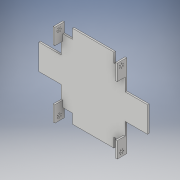
# Autodesk Inventor part: Gen2PlatePart
Saved by Autodesk Inventor 2017 (Build 210142000, 142)
## iProperties
Created: 2017-12-06
Part Number: Gen2PlatePart
Material: Generic
Document SubType Name: Modeling
Designer: User
Density: 1 g/cm^3
Appearance: Default
Author: User
Autodesk Inventor part; units mm, degrees
ref_plane "YZ Plane" through (0, 0, 0) normal (1, 0, 0) x (0, 1, 0)
ref_plane "XZ Plane" through (0, 0, 0) normal (0, 1, 0) x (-1, 0, 0)
ref_plane "XY Plane" through (0, 0, 0) normal (0, 0, 1) x (1, 0, 0)
sketch "Sketch1" plane through (0, 0, 0) normal (0, 0, 1) x (1, 0, 0)
  line L0 (0, 0) -> (254, 0)
  line L1 (254, 0) -> (254, 330.2)
  line L2 (254, 330.2) -> (0, 330.2)
  line L3 (0, 330.2) -> (0, 0)
  dimension "d0" = 254
  dimension "d1" = 330.2
  constraints: 8 end point, 2 parallel, 1 horizontal, 1 perpendicular
  measures "d0" distance of L2.end L1.end
  measures "d1" distance of L1.end L0.end
extrude "Extrusion1" add sketch "Sketch1" along normal blind 6.35
sketch "Sketch2" plane through (0, 0, 6.35) normal (0, 0, 1) x (1, 0, 0)
  point P0 (0, 0)
sketch "Sketch3" plane through (0, 0, 0) normal (-1, 0, 0) x (0, 0, 1)
  line L0 (0, 0) -> (0, 330.2) projected
  line L1 (0, 330.2) -> (-38.1, 330.2)
  line L2 (-38.1, 330.2) -> (38.1, 330.2)
  line L3 (38.1, 330.2) -> (38.1, 266.7)
  line L4 (38.1, 266.7) -> (-38.1, 266.7)
  line L5 (-38.1, 266.7) -> (-38.1, 330.2)
  line L6 (-38.1, 0) -> (38.1, 0)
  line L7 (38.1, 0) -> (38.1, 63.5)
  line L8 (38.1, 63.5) -> (-38.1, 63.5)
  line L9 (-38.1, 63.5) -> (-38.1, 0)
  dimension "d4" = 38.1
  dimension "d5" = 76.2
  dimension "d6" = 63.5
  dimension "d9" = 63.5
  constraints: 18 end point, 4 parallel, 3 horizontal, 2 perpendicular
  measures "d4" distance of L0.end L1.end
  measures "d5" distance of L3.end L4.end
  measures "d6" distance of L2.end L3.end
  measures "d9" distance of L7.end L6.end
extrude "Extrusion2" add sketch "Sketch3" against normal blind 6.35
sketch "Sketch4" plane through (6.35, 0, 0) normal (0, -1, 0) x (1, 0, 0)
  line L0 (0, -38.1) -> (0, 0) projected
  line L1 (247.65, 6.35) -> (0, 6.35) projected
  line L2 (0, 0) -> (38.1, 0)
  line L3 (38.1, 0) -> (38.1, 6.35)
  line L4 (38.1, 6.35) -> (0, 6.35)
  line L5 (0, 6.35) -> (0, 0)
  point P0 (-6.35, 0)
  dimension "d10" = 38.1
  constraints: 8 end point, 2 parallel, 1 horizontal, 1 perpendicular, 1 point on line
  measures "d10" distance of L4.end L3.end
extrude "Extrusion3" cut sketch "Sketch4" against normal blind 38.1
sketch "Sketch5" plane through (6.35, 330.2, 0) normal (0, 1, 0) x (1, 0, 0)
  line L0 (0, 0) -> (-6.35, 0) projected
  line L1 (0, -6.35) -> (38.1, -6.35) projected
  line L2 (0, 0) -> (38.1, 0)
  line L3 (38.1, 0) -> (38.1, -6.35)
  line L4 (38.1, -6.35) -> (0, -6.35)
  line L5 (0, -6.35) -> (0, 0)
  constraints: 8 end point, 2 parallel, 1 horizontal, 1 perpendicular
extrude "Extrusion4" cut sketch "Sketch5" against normal blind 38.1
sketch "Sketch6" plane through (254, 0, 0) normal (1, 0, 0) x (0, 0, -1)
  line L0 (38.1, 0) -> (-38.1, 0) projected
  line L1 (38.1, 63.5) -> (0, 63.5) projected
  line L2 (-38.1, 0) -> (38.1, 0)
  line L3 (38.1, 0) -> (38.1, 63.5)
  line L4 (38.1, 63.5) -> (-38.1, 63.5)
  line L5 (-38.1, 63.5) -> (-38.1, 0)
  line L6 (-38.1, 266.7) -> (-6.35, 266.7) projected
  line L7 (38.1, 330.2) -> (-38.1, 330.2) projected
  line L8 (-38.1, 266.7) -> (38.1, 266.7)
  line L9 (38.1, 266.7) -> (38.1, 330.2)
  line L10 (38.1, 330.2) -> (-38.1, 330.2)
  line L11 (-38.1, 330.2) -> (-38.1, 266.7)
  point P0 (0, 0)
  constraints: 16 end point, 4 parallel, 2 horizontal, 2 perpendicular
extrude "Extrusion5" add sketch "Sketch6" against normal blind 6.35
sketch "Sketch7" plane through (44.45, 330.2, 6.35) normal (0, 1, 0) x (1, 0, 0)
  line L0 (0, 0) -> (203.2, 0) projected
  line L1 (0, 6.35) -> (203.2, 6.35) projected
  line L2 (203.2, 0) -> (165.1, 0)
  line L3 (165.1, 0) -> (165.1, 6.35)
  line L4 (165.1, 6.35) -> (203.2, 6.35)
  line L5 (203.2, 6.35) -> (203.2, 0)
  point P0 (-44.45, 6.35)
  dimension "d17" = 38.1
  constraints: 8 end point, 2 parallel, 1 horizontal, 1 perpendicular, 1 point on line
  measures "d17" distance of L3.end L4.end
extrude "Extrusion6" cut sketch "Sketch7" against normal blind 38.1
sketch "Sketch8" plane through (44.45, 0, 0) normal (0, -1, 0) x (1, 0, 0)
  line L0 (209.55, 0) -> (203.2, 0) projected
  line L1 (0, 6.35) -> (203.2, 6.35) projected
  line L2 (203.2, 0) -> (165.1, 0)
  line L3 (165.1, 0) -> (165.1, 6.35)
  line L4 (165.1, 6.35) -> (203.2, 6.35)
  line L5 (203.2, 6.35) -> (203.2, 0)
  point P0 (-44.45, 0)
  dimension "d20" = 38.1
  constraints: 8 end point, 2 parallel, 1 horizontal, 1 perpendicular, 1 point on line
  measures "d20" distance of L3.end L4.end
extrude "Extrusion7" cut sketch "Sketch8" against normal blind 38.1
sketch "Sketch9" plane through (6.35, 0, 0) normal (1, 0, 0) x (0, 0, -1)
  line L0 (38.1, 0) -> (-38.1, 0) projected
  line L1 (-19.0903, 0) -> (-19.0903, 17.1196)
  line L2 (-19.0903, 0) -> (-1.9707, 0) construction
  line L3 (-38.1, 63.5) -> (-38.1, 0) projected
  line L4 (-38.1, 17.1196) -> (-20.955, 17.1196)
  line L5 (-38.1, 17.1196) -> (-20.955, 17.1196) construction
  circle A0 centre (-20.955, 17.1196) radius 3.4925
  point P0 (0, 0)
  dimension "d23" = 17.1196
  dimension "d24" = 90
  dimension "d25" = 17.145
  dimension "d26" = 0
  dimension "d27" = 6.985
  constraints: 8 end point, 2 equal length, 2 horizontal, 2 perpendicular, 2 point on line, 1 centre point, 1 coincident
  measures "d23" distance of L1.start L1.end
  measures "d24" angle of L2 L1
  measures "d25" distance of L4.start L4.end
  measures "d26" distance between parallel lines of L4 L5
  measures "d27" diameter of A0
extrude "Extrusion8" cut sketch "Sketch9" against normal blind 38.1 contours A0
sketch "Sketch10" plane through (6.35, 0, 0) normal (1, 0, 0) x (0, 0, -1)
  circle A0 centre (-20.955, 17.1196) radius 3.4925 projected
  circle A1 centre (-20.955, 17.1196) radius 8
  circle A2 centre (-20.955, 9.1196) radius 1.5875
  circle A3 centre (-14.0268, 13.1196) radius 1.5875
  circle A4 centre (-20.955, 17.1196) radius 8
  circle A5 centre (-14.0268, 21.1196) radius 1.5875
  circle A6 centre (-20.955, 17.1196) radius 8
  circle A7 centre (-20.955, 25.1196) radius 1.5875
  circle A8 centre (-20.955, 17.1196) radius 8
  circle A9 centre (-27.8832, 21.1196) radius 1.5875
  circle A10 centre (-20.955, 17.1196) radius 8
  circle A11 centre (-27.8832, 13.1196) radius 1.5875
  circle A12 centre (-20.955, 17.1196) radius 8
  point P0 (0, 0)
  point P1 (-28.955, 17.1196)
  point P2 (-24.955, 10.1914)
  point P3 (-16.955, 10.1914)
  point P4 (-12.955, 17.1196)
  point P5 (-16.955, 24.0478)
  point P6 (-24.955, 24.0478)
  dimension "d33" = 3.175
  dimension "d36" = 360
  constraints: 12 centre point, 12 point on circle, 9 coincident, 35 other
  measures "d33" diameter of A2
extrude "Extrusion9" cut sketch "Sketch10" against normal blind 38.1 contours A5 A1 | A1 A5 | A3 A1 | A1 A3 | A7 A1 | A1 A7 | A2 A1 | A1 A2 | A9 A1 | A1 A9 | A11 A1 | A1 A11
sketch "Sketch11" plane through (247.65, 0, 0) normal (-1, 0, 0) x (0, 0, 1)
  line L0 (38.1, 0) -> (38.1, 63.5) projected
  line L1 (38.1, 17.1196) -> (70.485, 17.1196) construction
  circle A0 centre (20.955, 17.1196) radius 3.4925
  circle A1 centre (20.955, 17.1196) radius 8.001
  line L2 (20.955, 17.1196) -> (31.4906, 17.1196)
  circle A2 centre (28.956, 17.1196) radius 1.5875
  circle A3 centre (24.9555, 24.0487) radius 1.5875
  circle A4 centre (20.955, 17.1196) radius 8.001
  circle A5 centre (16.9545, 24.0487) radius 1.5875
  circle A6 centre (20.955, 17.1196) radius 8.001
  circle A7 centre (12.954, 17.1196) radius 1.5875
  circle A8 centre (20.955, 17.1196) radius 8.001
  circle A9 centre (16.9545, 10.1905) radius 1.5875
  circle A10 centre (20.955, 17.1196) radius 8.001
  circle A11 centre (24.9555, 10.1905) radius 1.5875
  circle A12 centre (20.955, 17.1196) radius 8.001
  point P0 (0, 0)
  point P1 (20.955, 9.1186)
  point P2 (27.8841, 13.1191)
  point P3 (27.8841, 21.1201)
  point P4 (20.955, 25.1206)
  point P5 (14.0259, 21.1201)
  point P6 (14.0259, 13.1191)
  dimension "d44" = 16.002
  dimension "d41" = 17.145
  dimension "d43" = 6.985
  dimension "d81" = 3.175
  dimension "d84" = 360
  constraints: 7 centre point, 4 end point, 3 coincident, 2 point on line, 2 vertical alignment, 1 horizontal, 47 other
  measures "d41" distance of L1.start point (20.955, 17.12)
  measures "d43" diameter of A0
  measures "d81" diameter of A2
extrude "Extrusion10" cut sketch "Sketch11" against normal blind 25.4 contours A0 | L2 A2 A1 | L2 A2 A1 | A1 A2 L2 | A1 A2 L2 | A3 A1 | A1 A3 | A11 A1 | A1 A11 | A5 A1 | A1 A5 | A9 A1 | A1 A9 | A7 A1 | A1 A7
sketch "Sketch12" plane through (254, 63.5, 0) normal (1, 0, 0) x (0, 0, -1)
  line L0 (-38.1, 266.7) -> (-38.1, 203.2) projected
  line L1 (-38.1, 234.95) -> (-20.955, 234.95)
  line L2 (0, 228.6) -> (0, 266.7) projected
  line L3 (38.1, 266.7) -> (-38.1, 266.7) projected
  line L4 (-20.955, 266.7) -> (-20.955, 249.5804)
  line L5 (-20.955, 266.7) -> (-3.8354, 266.7) construction
  circle A0 centre (-20.955, 249.5804) radius 3.4925
  circle A1 centre (-20.955, 249.5804) radius 8.001
  line L6 (-20.955, 234.95) -> (-20.955, 230.7922)
  line L7 (-20.955, 249.5804) -> (-30.6683, 249.5804)
  line L8 (-6.35, 266.7) -> (-6.35, 228.6) projected
  circle A2 centre (-20.955, 257.5814) radius 1.5875
  circle A3 centre (-27.8841, 253.5809) radius 1.5875
  circle A4 centre (-20.955, 249.5804) radius 8.001
  circle A5 centre (-27.8841, 245.5799) radius 1.5875
  circle A6 centre (-20.955, 249.5804) radius 8.001
  circle A7 centre (-20.955, 241.5794) radius 1.5875
  circle A8 centre (-20.955, 249.5804) radius 8.001
  circle A9 centre (-14.0259, 245.5799) radius 1.5875
  circle A10 centre (-20.955, 249.5804) radius 8.001
  circle A11 centre (-14.0259, 253.5809) radius 1.5875
  circle A12 centre (-20.955, 249.5804) radius 8.001
  point P0 (0, -63.5)
  dimension "d56" = 16.002
  dimension "d52" = 17.145
  dimension "d53" = 17.1196
  dimension "d54" = 90
  dimension "d55" = 6.985
  dimension "d80" = 0
  dimension "d104" = 3.175
  dimension "d107" = 360
  constraints: 10 end point, 8 coincident, 7 centre point, 4 perpendicular, 2 point on line, 2 vertical alignment, 1 horizontal, 1 midpoint, 1 vertical, 47 other
  measures "d52" distance of L1.start L1.end
  measures "d53" distance of L4.start L4.end
  measures "d54" angle of L4 L5
  measures "d55" diameter of A0
  measures "d80" distance from line of L4.end L6
  measures "d104" diameter of A2
extrude "Extrusion11" cut sketch "Sketch12" against normal blind 25.4 contours A2 A1 L4 | L4 A1 A2 | A1 A2 L4 | L4 A2 A1 | A3 A1 | A1 A3 | A0 L7 L4 | L4 L7 A0 | A11 A1 | A1 A11 | A5 A1 | A1 A5 | A9 A1 | A1 A9 | A7 A1 | A1 A7
sketch "Sketch13" plane through (0, 63.5, 0) normal (-1, 0, 0) x (0, 0, 1)
  line L0 (-38.1, 266.7) -> (38.1, 266.7) projected
  line L1 (23.9735, 266.7) -> (41.0931, 266.7) construction
  line L2 (38.1, 249.5804) -> (20.955, 249.5804)
  line L3 (38.1, 249.5804) -> (55.245, 249.5804) construction
  circle A0 centre (20.955, -46.3804) radius 3.4925 projected
  line L4 (38.1, -63.5) -> (38.1, 0) projected
  circle A1 centre (20.955, 249.5804) radius 3.4925
  circle A2 centre (20.955, 249.5804) radius 8.001
  circle A3 centre (28.956, 249.5804) radius 1.5875
  circle A4 centre (24.9555, 256.5095) radius 1.5875
  circle A5 centre (20.955, 249.5804) radius 8.001
  circle A6 centre (16.9545, 256.5095) radius 1.5875
  circle A7 centre (20.955, 249.5804) radius 8.001
  circle A8 centre (12.954, 249.5804) radius 1.5875
  circle A9 centre (20.955, 249.5804) radius 8.001
  circle A10 centre (16.9545, 242.6513) radius 1.5875
  circle A11 centre (20.955, 249.5804) radius 8.001
  circle A12 centre (24.9555, 242.6513) radius 1.5875
  circle A13 centre (20.955, 249.5804) radius 8.001
  line L5 (38.1, 203.2) -> (6.35, 203.2) projected
  point P0 (0, -63.5)
  point P1 (20.9804, 257.5814)
  point P2 (14.0387, 253.6029)
  point P3 (14.0133, 245.6019)
  point P4 (20.9296, 241.5794)
  point P5 (27.8713, 245.5579)
  point P6 (27.8967, 253.5589)
  dimension "d67" = 17.145
  dimension "d68" = 180
  dimension "d69" = 17.145
  dimension "d70" = 6.985
  dimension "d71" = 6.985
  dimension "d72" = 16.002
  dimension "d92" = 3.175
  dimension "d95" = 360
  dimension "d134" = 46.3804
  constraints: 13 centre point, 12 point on circle, 6 end point, 3 horizontal, 2 coincident, 2 point on line, 1 collinear, 31 other
  measures "d67" distance of L2.start L2.end
  measures "d68" angle of L2 L3
  measures "d69" distance from line of A0.centre L4
  measures "d70" diameter of A0
  measures "d71" diameter of A1
  measures "d72" diameter of A2
  measures "d92" diameter of A3
  measures "d134" distance from line of L5 L2.end
extrude "Extrusion12" cut sketch "Sketch13" against normal blind 25.4 contours A3 A2 L2 | L2 A2 A3 | A2 A3 L2 | L2 A3 A2 | A4 A2 | A2 A4 | A12 A2 | A2 A12 | A6 A2 | A2 A6 | A10 A2 | A2 A10 | A8 A2 | A2 A8 | A1
sketch "Sketch14" plane through (254, 63.5, 0) normal (1, 0, 0) x (0, 0, -1)
  line L0 (0, -63.5) -> (0, 50.8)
  line L1 (0, 203.2) -> (0, 0) projected
  line L2 (38.1, 266.7) -> (-38.1, 266.7) projected
  line L3 (0, 266.7) -> (0, 165.1)
  line L4 (-6.35, 203.2) -> (-6.35, 0) projected
  line L5 (0, 50.8) -> (-6.35, 50.8)
  line L6 (-6.35, 241.3) -> (0, 241.3)
  line L7 (0, 241.3) -> (0, 50.8)
  line L8 (0, 266.7) -> (-6.35, 266.7) projected
  line L9 (0, 266.7) -> (0, 152.4)
  line L10 (0, 0) -> (0, 203.2) projected
  line L11 (-6.35, 0) -> (-6.35, 203.2) projected
  line L12 (0, 50.8) -> (-6.35, 50.8)
  line L13 (-6.35, 50.8) -> (-6.35, 152.4)
  line L14 (-6.35, 152.4) -> (0, 152.4)
  line L15 (0, 152.4) -> (0, 50.8)
  dimension "d109" = 114.3
  dimension "d137" = 114.3
  constraints: 20 end point, 5 point on line, 3 parallel, 2 horizontal, 1 midpoint, 1 perpendicular
  measures "d109" distance of L0.start L0.end
  measures "d137" distance of L3.start L9.end
sketch "Sketch15" plane through (0, 63.5, 0) normal (-1, 0, 0) x (0, 0, 1)
  line L0 (0, -63.5) -> (0, 38.1)
  line L1 (0, 0) -> (0, -25.4) projected
  line L2 (-38.1, 266.7) -> (38.1, 266.7) projected
  line L3 (0, 266.7) -> (0, 165.1)
  line L4 (0, 266.7) -> (0, 228.6) projected
  line L5 (6.35, 241.3) -> (6.35, 38.1) projected
  line L6 (0, 165.1) -> (6.35, 165.1)
  line L7 (6.35, 165.1) -> (6.35, 38.1)
  line L8 (6.35, 38.1) -> (0, 38.1)
  line L9 (0, 38.1) -> (0, 165.1)
  dimension "d113" = 101.6
  dimension "d114" = 101.6
  constraints: 12 end point, 2 collinear, 2 parallel, 1 horizontal, 1 midpoint, 1 perpendicular
  measures "d113" distance of L0.start L0.end
  measures "d114" distance of L3.start L3.end
extrude "Extrusion14" add sketch "Sketch15" along normal blind 88.9
thicken "Thicken1" operation add thickness 22.225 both sides no extend neighbours yes toward (0, 0, 1) faces at (251.8833, 287.8667, -38.1)
thicken "Thicken2" operation add thickness 22.225 both sides no extend neighbours yes toward (0, 0, 1) faces at (2.1167, 287.8667, -38.1)
thicken "Thicken3" operation add thickness 22.225 both sides no extend neighbours yes toward (0, 0, 1) faces at (2.1167, 42.3333, -38.1)
thicken "Thicken4" operation add thickness 22.225 both sides no extend neighbours yes toward (0, 0, 1) faces at (251.8833, 21.1667, -38.1)
sketch "Sketch16" plane through (247.65, 0, 0) normal (-1, 0, 0) x (0, 0, 1)
  point P0 (0, 0)
sketch "Sketch17" plane through (0, 0, 6.35) normal (0, 0, 1) x (1, 0, 0)
  point P0 (0, 0)
extrude "Extrusion15" add sketch "Sketch14" along normal blind 88.9
thicken "Thicken10" operation add thickness 12.7 both sides no extend neighbours yes toward (0, -1, 0) faces at (-29.6333, 228.6, 4.2333)
thicken "Thicken11" operation add thickness 12.7 both sides no extend neighbours yes toward (0, 1, 0) faces at (-29.6333, 101.6, 2.1167)
thicken "Thicken12" operation add thickness 15.875 both sides no extend neighbours yes toward (0, 0, 1) faces at (249.7667, 309.0333, -15.875)
thicken "Thicken13" operation add thickness 15.875 both sides no extend neighbours yes toward (0, 0, 1) faces at (4.2333, 287.8667, -15.875)
thicken "Thicken14" operation add thickness 15.875 both sides no extend neighbours yes toward (0, 0, 1) faces at (251.8833, 21.1667, -15.875)
thicken "Thicken15" operation add thickness 15.875 both sides no extend neighbours yes toward (0, 0, 1) faces at (2.1167, 42.3333, -15.875)
body "Solid1"
